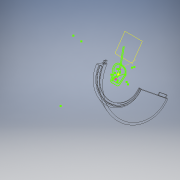
# Autodesk Inventor part: A1_V1_M2_dropArm_WOK_meso_tall_VIS_rt
Saved by Autodesk Inventor 2018 (Build 220112000, 112)
## iProperties
Created: 2018-04-20
Part Number: A1_V1_M2_dropArm_WOK_meso_tall_VIS_rt
Material: Generic
Document SubType Name: Modeling
Designer: McCormick Lab
Density: 1 g/cm^3
Appearance: Default
Author: McCormick Lab
Autodesk Inventor part; units mm, degrees
ref_plane "YZ Plane" through (0, 0, 0) normal (1, 0, 0) x (0, 1, 0)
ref_plane "XZ Plane" through (0, 0, 0) normal (0, 1, 0) x (-1, 0, 0)
ref_plane "XY Plane" through (0, 0, 0) normal (0, 0, 1) x (1, 0, 0)
sketch "Sketch68" plane through (0, 0, 0) normal (1, 0, 0) x (0, 1, 0)
  line L0 (1, 4.6737) -> (23, 4.6737) construction
  line L1 (7.0021, -2.9903) -> (-7.0029, -0.0135)
  line L2 (7.2385, 26.8729) -> (5.7713, 27.1847)
  line L3 (2.4565, 4.3755) -> (1, 4.6737)
  line L4 (5.7713, 27.1847) -> (1, 4.6737)
  line L5 (7.2385, 26.8729) -> (2.4565, 4.3755)
  point P0 (0, 0)
  point P1 (2.225, 5.1772)
  constraints: 12 end point, 1 horizontal
sketch "Sketch184" plane through (0, 0, 0) normal (1, 0, 0) x (0, 1, 0)
  arc A0 (-3.5, -3.0972) -> (0, -1.6204) centre (-4.281, 3.6397) ccw
  arc A1 (0, -1.6204) -> (2.2822, 2) centre (-4.3557, 3.6547) ccw
  arc A2 (2.2822, 2) -> (2.459, 4.3851) centre (-8.8285, 4.0231) ccw
  arc A3 (2.459, 4.3851) -> (2.3883, 6) centre (-72.7121, 1.9029) ccw
  line L0 (-3.5, -3.0972) -> (-3.5, -3.6807) projected
  arc A4 (2.3883, 6) -> (-3.5, -3.0972) centre (8.6947, -4.5362) ccw
  point P0 (0, 0)
  constraints: 10 point on circle, 5 centre point
ref_plane "Work Plane13" through (-1.8188, 14.8649, 21.2051) normal (0, 0.8198728, -0.5725457) x (1, 0, 0)
sketch "Sketch199" plane through (-1.8188, 14.8649, 21.2051) normal (0, 0.8198728, -0.5725457) x (1, 0, 0)
  arc A0 (-4.7396, 24.5206) -> (-5.4434, 21.3285) centre (-1.0506, 22.0335) ccw
  arc A1 (-3, 27) -> (-4.7396, 24.5206) centre (12.4104, 14.3381) ccw
  arc A2 (-2.529, 32.2114) -> (-3, 27) centre (13.6873, 28.1188) ccw
  arc A3 (-1.0506, 33.1641) -> (-2.529, 32.2114) centre (-1.0598, 31.555) ccw
  line L0 (-1.0506, 33.1641) -> (5.2457, 33.1641)
  arc A4 (6.5345, 31.555) -> (5.2457, 33.1641) centre (3.9319, 30.7911) ccw
  arc A5 (8.0214, 23.5206) -> (6.5345, 31.555) centre (-50.214, 16.898) ccw
  arc A6 (3.9319, 18.2442) -> (8.0214, 23.5206) centre (2.6688, 23.4462) ccw
  arc A7 (-5.4434, 21.3285) -> (-2.264, 17.7532) centre (-1.0506, 22.0335) ccw
  arc A8 (-2.264, 17.7532) -> (3.9319, 18.2442) centre (-0.0763, 29.4839) ccw
  point P0 (1.8188, 25.8963)
  constraints: 18 point on circle, 9 centre point, 2 end point, 1 concentric, 1 horizontal
ref_plane "Work Plane14" through (-1.8188, 14.8649, 21.2051) normal (0, 0.8198728, -0.5725457) x (1, 0, 0)
sketch "Sketch200" plane through (-1.8188, 14.8649, 21.2051) normal (0, 0.8198728, -0.5725457) x (1, 0, 0)
  arc A0 (-4.7396, 24.5206) -> (-5.4434, 21.3285) centre (-1.0506, 22.0335) ccw
  arc A1 (-3, 27) -> (-4.7396, 24.5206) centre (12.4104, 14.3381) ccw
  arc A2 (-2.529, 32.2114) -> (-3, 27) centre (13.6873, 28.1188) ccw
  arc A3 (-1.0506, 33.1641) -> (-2.529, 32.2114) centre (-1.0598, 31.555) ccw
  line L0 (-1.0506, 33.1641) -> (5.2457, 33.1641)
  arc A4 (6.5345, 31.555) -> (5.2457, 33.1641) centre (3.9319, 30.7911) ccw
  arc A5 (8.0214, 23.5206) -> (6.5345, 31.555) centre (-50.214, 16.898) ccw
  arc A6 (3.9319, 18.2442) -> (8.0214, 23.5206) centre (2.6688, 23.4462) ccw
  arc A7 (-5.4434, 21.3285) -> (-2.264, 17.7532) centre (-1.0506, 22.0335) ccw
  arc A8 (-2.264, 17.7532) -> (3.9319, 18.2442) centre (-0.0763, 29.4839) ccw
  point P0 (1.8188, 25.8963)
  constraints: 18 point on circle, 9 centre point, 2 end point, 1 concentric, 1 horizontal
ref_plane "Work Plane15" through (-1.8188, 14.8649, 21.2051) normal (0, 0.8198728, -0.5725457) x (1, 0, 0)
sketch "Sketch201" plane through (-1.8188, 14.8649, 21.2051) normal (0, 0.8198728, -0.5725457) x (1, 0, 0)
  arc A0 (-4.7396, 24.5206) -> (-5.4434, 21.3285) centre (-1.0506, 22.0335) ccw
  arc A1 (-3, 27) -> (-4.7396, 24.5206) centre (12.4104, 14.3381) ccw
  arc A2 (-2.529, 32.2114) -> (-3, 27) centre (13.6873, 28.1188) ccw
  arc A3 (-1.0506, 33.1641) -> (-2.529, 32.2114) centre (-1.0598, 31.555) ccw
  line L0 (-1.0506, 33.1641) -> (5.2457, 33.1641)
  arc A4 (6.5345, 31.555) -> (5.2457, 33.1641) centre (3.9319, 30.7911) ccw
  arc A5 (8.0214, 23.5206) -> (6.5345, 31.555) centre (-50.214, 16.898) ccw
  arc A6 (3.9319, 18.2442) -> (8.0214, 23.5206) centre (2.6688, 23.4462) ccw
  arc A7 (-2.264, 17.7532) -> (3.9319, 18.2442) centre (-0.0763, 29.4839) ccw
  arc A8 (-5.4434, 21.3285) -> (-2.264, 17.7532) centre (-1.0506, 22.0335) ccw
  arc A9 (-4.7396, 24.5206) -> (-5.4434, 21.3285) centre (-1.0506, 22.0335) ccw
  arc A10 (-3, 27) -> (-4.7396, 24.5206) centre (12.4104, 14.3381) ccw
  arc A11 (-2.529, 32.2114) -> (-3, 27) centre (13.6873, 28.1188) ccw
  arc A12 (-1.0506, 33.1641) -> (-2.529, 32.2114) centre (-1.0598, 31.555) ccw
  line L1 (-1.0506, 33.1641) -> (5.2457, 33.1641)
  arc A13 (6.5345, 31.555) -> (5.2457, 33.1641) centre (3.9319, 30.7911) ccw
  arc A14 (8.0214, 23.5206) -> (6.5345, 31.555) centre (-50.214, 16.898) ccw
  arc A15 (3.9319, 18.2442) -> (8.0214, 23.5206) centre (2.6688, 23.4462) ccw
  arc A16 (-2.264, 17.7532) -> (3.9319, 18.2442) centre (-0.0763, 29.4839) ccw
  arc A17 (-5.4434, 21.3285) -> (-2.264, 17.7532) centre (-1.0506, 22.0335) ccw
  arc A18 (-4.7396, 24.5206) -> (-5.4434, 21.3285) centre (-1.0506, 22.0335) ccw
  arc A19 (-3, 27) -> (-4.7396, 24.5206) centre (12.4104, 14.3381) ccw
  arc A20 (-2.529, 32.2114) -> (-3, 27) centre (13.6873, 28.1188) ccw
  arc A21 (-1.0506, 33.1641) -> (-2.529, 32.2114) centre (-1.0598, 31.555) ccw
  line L2 (-1.0506, 33.1641) -> (5.2457, 33.1641)
  arc A22 (6.5345, 31.555) -> (5.2457, 33.1641) centre (3.9319, 30.7911) ccw
  arc A23 (8.0214, 23.5206) -> (6.5345, 31.555) centre (-50.214, 16.898) ccw
  arc A24 (3.9319, 18.2442) -> (8.0214, 23.5206) centre (2.6688, 23.4462) ccw
  arc A25 (-2.264, 17.7532) -> (3.9319, 18.2442) centre (-0.0763, 29.4839) ccw
  arc A26 (-5.4434, 21.3285) -> (-2.264, 17.7532) centre (-1.0506, 22.0335) ccw
  arc A27 (-2.529, 32.2114) -> (-3, 27) centre (13.6873, 28.1188) ccw
  arc A28 (-3, 27) -> (-4.7396, 24.5206) centre (12.4104, 14.3381) ccw
  arc A29 (-4.7396, 24.5206) -> (-5.4434, 21.3285) centre (-1.0506, 22.0335) ccw
  arc A30 (-5.4434, 21.3285) -> (-2.264, 17.7532) centre (-1.0506, 22.0335) ccw
  arc A31 (-2.264, 17.7532) -> (3.9319, 18.2442) centre (-0.0763, 29.4839) ccw
  arc A32 (3.9319, 18.2442) -> (8.0214, 23.5206) centre (2.6688, 23.4462) ccw
  arc A33 (8.0214, 23.5206) -> (6.5345, 31.555) centre (-50.214, 16.898) ccw
  arc A34 (6.5345, 31.555) -> (5.2457, 33.1641) centre (3.9319, 30.7911) ccw
  line L3 (-1.0506, 33.1641) -> (5.2457, 33.1641)
  arc A35 (-1.0506, 33.1641) -> (-2.529, 32.2114) centre (-1.0598, 31.555) ccw
  arc A36 (-3.4348, 34.2537) -> (-4, 28) centre (16.0247, 29.3425) ccw
  arc A37 (-4, 28) -> (-6.0875, 25.0247) centre (14.4925, 12.8057) ccw
  arc A38 (-3.1168, 16.9038) -> (4.3183, 17.4931) centre (-0.4915, 30.9807) ccw
  arc A39 (4.3183, 17.4931) -> (9.2257, 23.8247) centre (2.8025, 23.7355) ccw
  arc A40 (9.2257, 23.8247) -> (7.4414, 33.4659) centre (-60.6567, 15.8776) ccw
  arc A41 (7.4414, 33.4659) -> (5.8948, 35.3969) centre (4.3183, 32.5493) ccw
  line L4 (-1.6607, 35.3969) -> (5.8948, 35.3969)
  arc A42 (-1.6607, 35.3969) -> (-3.4348, 34.2537) centre (-1.6718, 33.4659) ccw
  arc A43 (-6.0875, 25.0247) -> (-6.9321, 21.1943) centre (-1.6607, 22.0403) ccw
  arc A44 (-6.9321, 21.1943) -> (-3.1168, 16.9038) centre (-1.6607, 22.0403) ccw
  point P0 (1.8188, 25.8963)
  constraints: 90 point on circle, 45 centre point, 10 end point, 5 horizontal, 4 concentric
sketch "Sketch213" plane through (0, 0, 0) normal (1, 0, 0) x (0, 1, 0)
  line L0 (13.3414, -11.8728) -> (-10.8201, 5)
  line L1 (46.9769, 13.1952) -> (16.4024, 18.5466)
  line L2 (-15.4661, -26.0463) -> (-0.3893, -51.1005)
  line L3 (-0.3893, -51.1005) -> (1.9473, -49.7476)
  line L4 (46.9769, 13.1952) -> (46.7355, 11.8161)
  line L5 (1.9473, -49.7476) -> (-11.7207, -26.1425)
  line L6 (-11.7207, -26.1425) -> (-10, -24)
  line L7 (-10, -24) -> (-10.853, -23.4043)
  line L8 (46.7355, 11.8161) -> (18.2275, 16.8059)
  line L9 (18.2275, 16.8059) -> (17, 15)
  line L10 (17, 15) -> (16.3637, 15.4444)
  line L11 (16.3637, 15.4444) -> (17.062, 16.4444)
  line L12 (17.062, 16.4444) -> (17.3561, 17.7094)
  line L13 (17.3561, 17.7094) -> (16.3637, 17.6698)
  line L14 (16.3637, 17.6698) -> (16.4024, 18.5466)
  line L15 (-10.853, -23.4043) -> (-11.9333, -25.0763)
  line L16 (-11.9333, -25.0763) -> (-13.146, -25.8811)
  line L17 (-13.146, -25.8811) -> (-12.9536, -24.5344)
  line L18 (-12.9536, -24.5344) -> (-15.4661, -26.0463)
  point P0 (0, 0)
  point P1 (3.3399, -2.2736)
  point P2 (-1.2043, -8.7808)
  dimension "d600" = 2.7
  dimension "d601" = 1.4
  dimension "d603" = 1.265
  constraints: 38 end point
  measures "d600" distance of L2.end L3.end
  measures "d601" distance of L1.start L4.end
  measures "d603" vertical distance of L12.end L11.end
revolve "Revolution6" add sketch "Sketch213" angle 180 mid plane about axis through (0, 13.3414, -11.8728) along (0, -0.8198728, 0.5725457) contours L18 L17 L16 L15 L7 L6 L5 L3 L2
sketch "Sketch214" plane through (-28.1141, 0.6305, -2.9963) normal (0, 0.5725457, 0.8198728) x (0.9133048, 0.3339151, -0.2331846)
  line L0 (71.2508, -4.0445) -> (70.3985, -3.0629)
  line L1 (70.3985, -3.0629) -> (64.3578, -8.3078)
  line L2 (71.2508, -4.0445) -> (65.2101, -9.2894)
  line L3 (64.3578, -8.3078) -> (65.2101, -9.2894)
  line L4 (2.6996, 29.2863) -> (0, 29.2408) projected
  line L5 (3.1595, 2.0136) -> (2.6996, 29.2863) projected
  line L6 (0, 29.2408) -> (0, 0) projected
  line L7 (0.7, 27.3772) -> (2, 27.3772)
  line L8 (0.7, 27.3772) -> (0.7, 19.3772)
  line L9 (2, 27.3772) -> (2, 19.3772)
  line L10 (0.7, 19.3772) -> (2, 19.3772)
  line L11 (51.3534, -22.9004) -> (73.1067, -3.3602) projected
  line L12 (73.1067, -3.3602) -> (71.3365, -1.3215) projected
  line L13 (71.3365, -1.3215) -> (50.7401, -19.2043) projected
  point P0 (24.7675, -13.4891)
  dimension "d606" = 8
  dimension "d625" = 90
  dimension "d626" = 0.7
  dimension "d630" = 1.3
  dimension "d635" = 0.7
  dimension "d637" = 1.85
  constraints: 16 end point, 2 vertical, 1 horizontal
  measures "d606" distance between parallel lines of L3 L0
  measures "d625" angle of L9 L7
  measures "d626" distance between parallel lines of L6 L8
  measures "d630" distance between parallel lines of L1 L2
  measures "d635" distance between parallel lines of L13 L1
  measures "d637" distance between parallel lines of L0 L12
extrude "Extrusion162" add sketch "Sketch214" along normal blind 3
body "Solid2"
